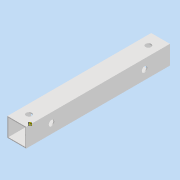
# Autodesk Inventor part: 4_barra
Saved by Autodesk Inventor 2020 (Build 240168000, 168)
## iProperties
Created: 2019-10-11
Part Number: 4_barra
Material: Generico
Document SubType Name: Modeling
Designer: socci
Density: 1 g/cm^3
Appearance: Default
Author: socci
Autodesk Inventor part; units mm, degrees
ref_plane "YZ Plane" through (0, 0, 0) normal (1, 0, 0) x (0, 1, 0)
ref_plane "XZ Plane" through (0, 0, 0) normal (0, 1, 0) x (-1, 0, 0)
ref_plane "XY Plane" through (0, 0, 0) normal (0, 0, 1) x (1, 0, 0)
sketch "Schizzo1" plane through (0, 0, 0) normal (0, 0, 1) x (1, 0, 0)
  line L0 (10, -10) -> (-10, -10)
  line L1 (-10, -10) -> (-10, 10)
  line L2 (-10, 10) -> (10, 10)
  line L3 (10, 10) -> (10, -10)
  line L4 (9, 9) -> (-9, 9)
  line L5 (-9, 9) -> (-9, -9)
  line L6 (-9, -9) -> (9, -9)
  line L7 (9, -9) -> (9, 9)
  point P0 (0, 0)
  point P1 (0, 0)
  dimension "d0" = 20
  dimension "d1" = 1
  constraints: 16 end point, 1 coincident, 12 other
  measures "d0" distance of L1.end L2.end
  measures "d1" distance between parallel lines of L2 L4
extrude "Estrusione1" add sketch "Schizzo1" against normal blind 153
sketch "Schizzo8" plane through (10, -10, 0) normal (1, 0, 0) x (0, 0, -1)
  circle A0 centre (126, 10) radius 2.75
  circle A1 centre (27, 10) radius 2.95
  circle A2 centre (126, 10) radius 2.75
  circle A3 centre (27, 10) radius 2.95
  point P0 (0, 10)
  constraints: 4 centre point, 2 coincident, 2 concentric, 4 other
hole "Foro7" at (10, 0, -126) at (10, 0, -27) direction (-1, 0, 0) diameter 5.9 end through all clearance for "Vite a testa piana" size "M5" standard "ANSI - Profilo M Metrico"
sketch "Schizzo9" plane through (-10, 10, 0) normal (0, 1, 0) x (1, 0, 0)
  circle A0 centre (10, 13) radius 2.95
  circle A1 centre (10, 140) radius 2.75
  circle A2 centre (10, 13) radius 2.95
  circle A3 centre (10, 140) radius 2.75
  point P0 (10, 0)
  constraints: 4 centre point, 2 coincident, 2 concentric, 4 other
hole "Foro8" at (0, 10, -13) at (0, 10, -140) direction (0, -1, 0) diameter 5.9 end through all clearance for "Vite a testa piana" size "M5" standard "ANSI - Profilo M Metrico"
